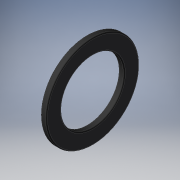
# Autodesk Inventor part: 51107 Shaft washer
Saved by Autodesk Inventor 2019 (Build 230136000, 136)
## iProperties
Created: 2023-07-26
Part Number: 51107 Shaft washer
Material: Generic
Catalog Web Link: www.cadenas.de
Description: With flat seet SW-
Vendor: NSK_RB
Document SubType Name: Modeling
Designer: psAdmin
Manufacturer: NSK_RB
Mass: 3.74339 g
Surface Area: 31.084 cm^2
Volume: 3.74339 cm^3
Density: 1 g/cm^3
Appearance: PSOLRGB-175-175-175
Category: PARTsolutions
Company: NSK_RB
Title: 51107 Shaft washer
Author: Cadenas PARTsolutions
PSOL_IDENT_0: {$CADENAS_DATA/23d-libs/nsk_rb/roller_bearings/thrust_bearings/single_direction_tbb/with_flat_seet_s
PSOL_IDENT_1: w.prj},189 {VTYP=3D},{NB=51107 Shaft washer},{LINA=51107 Shaft washer},{NN=With flat seet SW},{DATE=
PSOL_IDENT_2: 27.09.2022 23:23:10},{GEOMDATE=23.08.2022 10:45:55},{VERSION=},{LINEID=6430},{WBVAR=},{WBNUMERIC=}
PSOL_IDENT_3: {NB=51107 Shaft washer},{LINA=51107 Shaft washer},{KT=DUMMY},{IDNR=},{STAN=},{NO=19},{ORDER=51107},{
PSOL_IDENT_4: SD=35},{D=52},{T=12},{T3=0.0},{T4=0},{SR=0.6},{CAN=22100},{COAN=49500},{CA=2250},{COA=5050},{GRE=400
PSOL_IDENT_5: 0},{OIL=6000},{SD1=52},{D1=37},{D2=0},{D3=0},{SB=0.0},{A=0.0},{R=0},{SDA=45},{DA=42},{SRA=0.6},{MASS=
PSOL_IDENT_6: 0.081},{N=10},{DIST=2.133}
NB: 51107 Shaft washer
NN: With flat seet SW
NBSYN: $ORDER. Shaft washer
LINA: 51107 Shaft washer
CATALOG: NSK Rolling Bearing
NO: 19
ORDER: 51107
SD: 35
D: 52
T: 12
T3: 0
T4: 0
SR: 0.6
CAN: 22100
COAN: 49500
CA: 2250
COA: 5050
GRE: 4000
OIL: 6000
SD1: 52
D1: 37
D2: 0
D3: 0
SB: 0
A: 0
R: 0
SDA: 45
DA: 42
SRA: 0.6
MASS: 0.081
N: 10
SUPPLIER: NSK_RB
ARTICLENO: 51107 Shaft washer
BOMINFO: 51107 Shaft washer
CREATOR: CADENAS GmbH
Autodesk Inventor part; units mm, degrees
ref_plane "YZ Plane" through (0, 0, 0) normal (1, 0, 0) x (0, 1, 0)
ref_plane "XZ Plane" through (0, 0, 0) normal (0, 1, 0) x (-1, 0, 0)
ref_plane "XY Plane" through (0, 0, 0) normal (0, 0, 1) x (1, 0, 0)
sketch "Sketch_1" plane through (0, 0, 0) normal (0, 0, 1) x (1, 0, 0)
  line L0 (3.3333, 0) -> (0, 0)
  arc A0 (0, 20.8756) -> (0, 23.6244) centre (-2.6667, 22.25) ccw
  line L1 (0, 20.8756) -> (0, 18.1)
  arc A1 (0, 18.1) -> (0.6, 17.5) centre (0.6, 18.1) ccw
  line L2 (0.6, 17.5) -> (2.7333, 17.5)
  arc A2 (2.7333, 17.5) -> (3.3333, 18.1) centre (2.7333, 18.1) ccw
  line L3 (3.3333, 18.1) -> (3.3333, 25.4)
  arc A3 (3.3333, 25.4) -> (2.7333, 26) centre (2.7333, 25.4) ccw
  line L4 (2.7333, 26) -> (0.6, 26)
  arc A4 (0.6, 26) -> (0, 25.4) centre (0.6, 25.4) ccw
  line L5 (0, 25.4) -> (0, 23.6244)
  constraints: 12 end point, 10 point on circle, 5 centre point
revolve "Revolution1" add sketch "Sketch_1" angle 360 about axis through (3.3333, 0, 0) along (1, 0, 0)
ref_plane "SW_HW_XY" through (-8.6667, 0, 0) normal (1, 0, 0) x (0, 0, -1)
ref_plane "SW_HW_YZ" through (-8.6667, 0, 0) normal (0, 0, -1) x (0, 1, 0)
ref_plane "SW_HW_ZX" through (-8.6667, 0, 0) normal (0, 1, 0) x (1, 0, 0)
body "Solid1"
